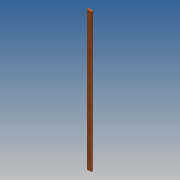
# Autodesk Inventor part: 2p2psv
Saved by Autodesk Inventor 2014 SP1 (Build 180222100, 222)
## iProperties
Created: 2013-09-03
Part Number: 2p2psv
Material: Wood (Cherry)
Document SubType Name: Modeling
Designer: David DeBoer
Mass: 3352.84 g
Surface Area: 5127.86 cm^2
Volume: 6705.68 cm^3
Density: 0.5 g/cm^3
Description: Pole stand vertical support
Appearance: Cherry - Natural Low Gloss
Author: Dave
Autodesk Inventor part; units mm, degrees
ref_plane "YZ Plane" through (0, 0, 0) normal (1, 0, 0) x (0, 1, 0)
ref_plane "XZ Plane" through (0, 0, 0) normal (0, 1, 0) x (-1, 0, 0)
ref_plane "XY Plane" through (0, 0, 0) normal (0, 0, 1) x (1, 0, 0)
sketch "Sketch1" plane through (0, 0, 0) normal (0, 1, 0) x (-1, 0, 0)
  line L0 (0, 0) -> (88.9, 0)
  line L1 (88.9, 0) -> (88.9, 38.1)
  line L2 (88.9, 38.1) -> (0, 38.1)
  line L3 (0, 38.1) -> (0, 0)
  dimension "d0" = 88.9
  dimension "d1" = 38.1
  constraints: 8 end point, 2 parallel, 1 horizontal, 1 perpendicular
  measures "d0" distance of L0.start L0.end
  measures "d1" distance of L2.end L0.start
extrude "Extrusion1" add sketch "Sketch1" along normal blind 2794
sketch "Sketch3" plane through (-88.9, 0, 38.1) normal (0, 0, 1) x (1, 0, 0)
  line L0 (0, 0) -> (88.9, 0) projected
  line L1 (0, 0) -> (0, 2794) projected
  circle A0 centre (25.4, 101.6) radius 5.7238
  circle A1 centre (63.5, 101.6) radius 5.7238
  circle A2 centre (25.4, 609.6) radius 5.7238
  circle A3 centre (63.5, 609.6) radius 5.7238
  dimension "d28" = 101.6
  dimension "d29" = 25.4
  dimension "d32" = 38.1
  dimension "d35" = 508
  constraints: 4 centre point, 1 horizontal, 1 vertical, 6 other
  measures "d28" distance from line of L0 A0.centre
  measures "d29" distance from line of A0.centre L1
  measures "d32" distance of A0.centre A1.centre
  measures "d35" distance of A0.centre A2.centre
hole "rimArm" at (-63.5, 609.6, 38.1) at (-25.4, 609.6, 38.1) at (-63.5, 101.6, 38.1) at (-25.4, 101.6, 38.1) direction (0, 0, -1) diameter 6.35 end through all
sketch "Sketch4" plane through (-88.9, 0, 38.1) normal (0, 0, 1) x (1, 0, 0)
  line L0 (0, 2794) -> (88.9, 2794) projected
  line L1 (0, 0) -> (0, 2794) projected
  circle A0 centre (25.4, 2774.95) radius 4.8454
  circle A1 centre (63.5, 2774.95) radius 4.8454
  circle A2 centre (25.4, 2139.95) radius 4.8454
  circle A3 centre (63.5, 2139.95) radius 4.8454
  dimension "d45" = 19.05
  dimension "d48" = 38.1
  dimension "d51" = 635
  constraints: 4 centre point, 1 horizontal, 1 vertical, 6 other
  measures "d45" distance from line of A0.centre L0
  measures "d48" distance of A0.centre A1.centre
  measures "d51" distance of A0.centre A2.centre
hole "screenArm" at (-63.5, 2774.95, 38.1) at (-25.4, 2774.95, 38.1) at (-25.4, 2139.95, 38.1) at (-63.5, 2139.95, 38.1) direction (0, 0, -1) diameter 6.7564 end through all clearance for "Flat Head Machine Screw (82)" size "1/4" standard "Ansi Unified Screw Threads"
sketch "Sketch5" plane through (-88.9, 0, 38.1) normal (0, 0, 1) x (1, 0, 0)
  line L0 (0, 0) -> (88.9, 0) projected
  line L1 (0, 2794) -> (88.9, 2794) projected
  circle A0 centre (44.45, 2667) radius 8.4367
  circle A1 centre (44.45, 1651) radius 12.5456
  circle A2 centre (44.45, 457.2) radius 11.5895
  dimension "d61" = 127
  dimension "d62" = 457.2
  dimension "d70" = 1651
  constraints: 3 centre point
  measures "d61" distance from line of L1 A0.centre
  measures "d62" distance from line of L0 A2.centre
  measures "d70" distance from line of L0 A1.centre
hole "poleAttach" at (-44.45, 2667, 38.1) at (-44.45, 1651, 38.1) at (-44.45, 457.2, 38.1) direction (0, 0, -1) diameter 10.0838 end through all clearance for "Flat Head Machine Screw (82)" size "3/8" standard "Ansi Unified Screw Threads"
body "Solid1"
